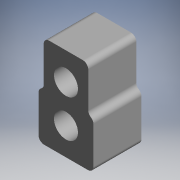
# Autodesk Inventor part: Tplug
Saved by Autodesk Inventor 2019 (Build 230136000, 136)
## iProperties
Part Number: Tplug
Material: Generic
Document SubType Name: Modeling
Designer: Jorge
Appearance: Default
Author: Jorge
Autodesk Inventor part; units mm, degrees
ref_plane "YZ Plane" through (0, 0, 0) normal (1, 0, 0) x (0, 1, 0)
ref_plane "XZ Plane" through (0, 0, 0) normal (0, 1, 0) x (-1, 0, 0)
ref_plane "XY Plane" through (0, 0, 0) normal (0, 0, 1) x (1, 0, 0)
sketch "Sketch1" plane through (0, 0, 0) normal (0, 0, 1) x (1, 0, 0)
  circle A0 centre (4, 9.5) radius 1.75
  circle A1 centre (4, 4) radius 1.75
  line L0 (4, 9.5) -> (4, 4) construction
  line L1 (0.75, 6.75) -> (0.75, 13.5)
  line L2 (0.75, 13.5) -> (7.25, 13.5)
  line L3 (7.25, 13.5) -> (7.25, 6.75)
  line L4 (0, 6.75) -> (0, 0)
  line L5 (0, 0) -> (8, 0)
  line L6 (8, 0) -> (8, 6.75)
  line L7 (0, 6.75) -> (0.75, 6.75)
  line L8 (7.25, 6.75) -> (8, 6.75)
  line L9 (0.75, 6.75) -> (7.25, 6.75) construction
  line L10 (4, 4) -> (4, 0) construction
  line L11 (4, 9.5) -> (4, 13.5) construction
  point P0 (4, 6.75)
  dimension "d0" = 3.5
  dimension "d1" = 3.5
  dimension "d2" = 5.5
  dimension "d3" = 6.5
  dimension "d4" = 8
  dimension "d5" = 13.5
  constraints: 24 end point, 4 midpoint, 4 perpendicular, 3 horizontal, 3 vertical, 2 centre point, 2 collinear, 1 coincident, 2 other
  measures "d0" diameter of A0
  measures "d1" diameter of A1
  measures "d2" distance of L0.start L0.end
  measures "d3" distance of L1.end L2.end
  measures "d4" distance of L4.end L5.end
  measures "d5" distance between parallel lines of L5 L2
extrude "Extrusion1" add sketch "Sketch1" along normal blind 7
fillet "Fillet1" radius 0.8 8 edges at (7.25, 13.5, 3.5) (0.75, 13.5, 3.5) (8, 0, 3.5) (0, 0, 3.5) (0.75, 6.75, 3.5) (0, 6.75, 3.5) (8, 6.75, 3.5) (7.25, 6.75, 3.5)
body "Solid1"
